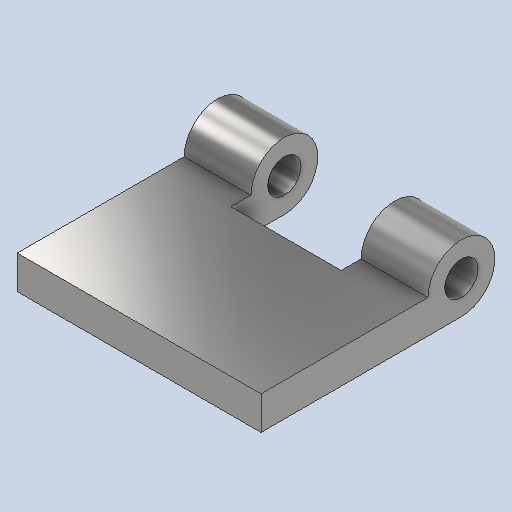
# Autodesk Inventor part: hinge 1
Saved by Autodesk Inventor 2022 (Build 260153000, 153)
## iProperties
Created: 2022-04-11
Part Number: hinge 1
Material: Stainless Steel
Document SubType Name: Modeling
Designer: MacBook
Density: 8 g/cm^3
Appearance: Semi-Polished
Author: MacBook
Autodesk Inventor part; units mm, degrees
ref_plane "YZ Plane" through (0, 0, 0) normal (1, 0, 0) x (0, 1, 0)
ref_plane "XZ Plane" through (0, 0, 0) normal (0, 1, 0) x (-1, 0, 0)
ref_plane "XY Plane" through (0, 0, 0) normal (0, 0, 1) x (1, 0, 0)
sketch "Sketch1" plane through (0, 0, 0) normal (0, 1, 0) x (-1, 0, 0)
  line L0 (-18.2563, -12.5) -> (18.2563, -12.5)
  line L1 (18.2563, -12.5) -> (18.2563, 12.5)
  line L2 (18.2563, 12.5) -> (-18.2563, 12.5)
  line L3 (-18.2563, 12.5) -> (-18.2563, -12.5)
  line L4 (-18.2563, -12.5) -> (18.2563, 12.5) construction
  line L5 (18.2563, -12.5) -> (-18.2563, 12.5) construction
  point P0 (0, 0)
  dimension "d0" = 36.5125
  dimension "d1" = 25
  constraints: 12 end point, 2 midpoint, 2 parallel, 1 horizontal, 1 perpendicular
  measures "d0" distance between parallel lines of L3 L1
  measures "d1" distance between parallel lines of L0 L2
extrude "Extrusion1" add sketch "Sketch1" against normal blind 5
sketch "Sketch2" plane through (18.2563, 0, 12.5) normal (1, 0, 0) x (0, 0, -1)
  line L0 (25, 0) -> (25, -5) projected
  circle A0 centre (30, 0) radius 5
  line L1 (25, -5) -> (0, -5) projected
  line L2 (25, -5) -> (30, -5)
  line L3 (30, -5) -> (30, 0)
  line L4 (30, 0) -> (25, 0)
  line L5 (25, 0) -> (25, -5)
  point P0 (12.5, 0)
  dimension "d4" = 5
  dimension "d5" = 5
  constraints: 8 end point, 2 parallel, 1 horizontal, 1 perpendicular, 3 other
  measures "d4" distance of L0.start L3.end
  measures "d5" distance from line of L1 L3.end
extrude "Extrusion2" add sketch "Sketch2" against normal blind 36.513
sketch "Sketch3" plane through (18.2563, -5, 12.5) normal (1, 0, 0) x (0, 0, -1)
  circle A0 centre (30, 5) radius 2.5
  line L0 (0, 5) -> (25, 5) projected
  point P0 (12.5, 5)
  dimension "d8" = 0
  dimension "d9" = 5
  dimension "d10" = 5
  constraints: 1 centre point
  measures "d8" distance from line of L0 A0.centre
  measures "d9" distance of L0.end A0.centre
  measures "d10" diameter of A0
extrude "Extrusion3" cut sketch "Sketch3" against normal blind 36.513
sketch "Sketch4" plane through (0, -5, 0) normal (0, -1, 0) x (1, 0, 0)
  line L0 (18.2563, -12.5) -> (-18.2563, -12.5) projected
  line L1 (18.2563, -22.5) -> (-18.2567, -22.5) projected
  line L2 (8.2563, -12.5) -> (-8.2568, -12.5)
  line L3 (-8.2568, -12.5) -> (-8.2567, -22.5)
  line L4 (-8.2567, -22.5) -> (8.2563, -22.5)
  line L5 (8.2563, -22.5) -> (8.2563, -12.5)
  line L6 (18.2563, -22.5) -> (18.2563, -12.5) projected
  line L7 (-18.2567, -12.5) -> (-18.2567, -22.5) projected
  line L8 (8.2563, -12.5) -> (-8.2567, -12.5)
  line L9 (-8.2567, -12.5) -> (-8.2567, -9.5)
  line L10 (-8.2567, -9.5) -> (8.2562, -9.5)
  line L11 (8.2562, -9.5) -> (8.2563, -12.5)
  point P0 (0, 0)
  point P1 (18.2563, -17.5)
  point P2 (-18.2567, -17.5)
  point P3 (8.2562, -11)
  dimension "d13" = 10
  dimension "d14" = 10
  dimension "d15" = 3
  dimension "d16" = 16.513
  constraints: 16 end point, 4 parallel, 2 horizontal, 2 perpendicular, 2 point on line, 1 midpoint
  measures "d13" distance between parallel lines of L6 L5
  measures "d14" distance between parallel lines of L7 L3
  measures "d15" distance between parallel lines of L0 L10
  measures "d16" distance from line of point (8.256, -11) L9
extrude "Extrusion4" cut sketch "Sketch4" against normal blind 36.513 contours L5 L1 L3 L0 | L0 L9 L10 L11
body "Solid1"
